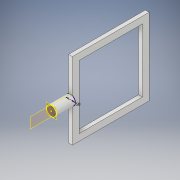
# Autodesk Inventor part: raquetteEsquisse
Saved by Autodesk Inventor 2019 (Build 230136000, 136)
## iProperties
Created: 2019-06-07
Part Number: raquetteEsquisse
Material: Plastique ABS
Document SubType Name: Modeling
Designer: tmayet
Mass: 1499.58 g
Surface Area: 1939.98 cm^2
Volume: 1414.7 cm^3
Density: 1.06 g/cm^3
Appearance: Lisse - Blanc
Author: tmayet
Autodesk Inventor part; units mm, degrees
ref_plane "YZ Plane" through (0, 0, 0) normal (1, 0, 0) x (0, 1, 0)
ref_plane "XZ Plane" through (0, 0, 0) normal (0, 1, 0) x (-1, 0, 0)
ref_plane "XY Plane" through (0, 0, 0) normal (0, 0, 1) x (1, 0, 0)
sketch "Esquisse1" plane through (0, 0, 0) normal (0, 0, 1) x (1, 0, 0)
  circle A0 centre (0, 0) radius 25
  point P0 (0, -25)
  point P1 (0, 25)
  dimension "d0" = 50
  constraints: 2 point on circle, 1 centre point, 1 coincident
  measures "d0" diameter of A0
extrude "Extrusion1" add sketch "Esquisse1" along normal blind 200
sketch "Esquisse2" plane through (0, 0, 0) normal (0, 0, -1) x (-1, 0, 0)
  point P0 (0, 0)
sketch "Esquisse3" plane through (0, 0, 200) normal (0, 0, 1) x (1, 0, 0)
  circle A0 centre (0, 0) radius 25 projected
  point P0 (0, -25)
  constraints: 1 vertical alignment, 1 other
ref_plane "Plan de construction1" through (0, -25, 0) normal (1, 0, 0) x (0, 1, 0)
sketch "Esquisse4" plane through (0, -25, 0) normal (1, 0, 0) x (0, 1, 0)
  line L0 (-175, -400) -> (225, -400)
  line L1 (225, -400) -> (225, 0)
  line L2 (225, 0) -> (-175, 0)
  line L3 (-175, 0) -> (-175, -400)
  line L4 (0, 0) -> (50, 0) projected
  line L5 (-140, -365) -> (190, -365)
  line L6 (190, -365) -> (190, -35)
  line L7 (190, -35) -> (-140, -35)
  line L8 (-140, -35) -> (-140, -365)
  point P0 (25, 0)
  dimension "d3" = 0
  dimension "d4" = 400
  dimension "d5" = 400
  dimension "d6" = 200
  dimension "d7" = 330
  dimension "d8" = 330
  dimension "d9" = 35
  dimension "d10" = 35
  constraints: 16 end point, 4 parallel, 2 horizontal, 2 perpendicular
  measures "d3" distance between parallel lines of L4 L2
  measures "d4" distance between parallel lines of L1 L3
  measures "d5" distance of L2.end L0.start
  measures "d6" distance from line of L3 point (25, 0)
  measures "d7" distance of L5.start L5.end
  measures "d8" distance of L7.end L5.start
  measures "d9" distance between parallel lines of L0 L5
  measures "d10" distance between parallel lines of L3 L8
extrude "Extrusion2" add sketch "Esquisse4" along normal mid plane 20
ref_plane "Plan de construction2" through (0, 0, 100) normal (0, 0, 1) x (1, 0, 0)
sketch "Esquisse5" plane through (0, 0, 100) normal (0, 0, 1) x (1, 0, 0)
  circle A0 centre (0, 0) radius 25 projected
equation "\"d6\" = 0.5 * d4"
equation "\"d9\" = -0.5 * d8 + 0.5 * d5"
equation "\"d10\" = -0.5 * d8 + 0.5 * d5"
